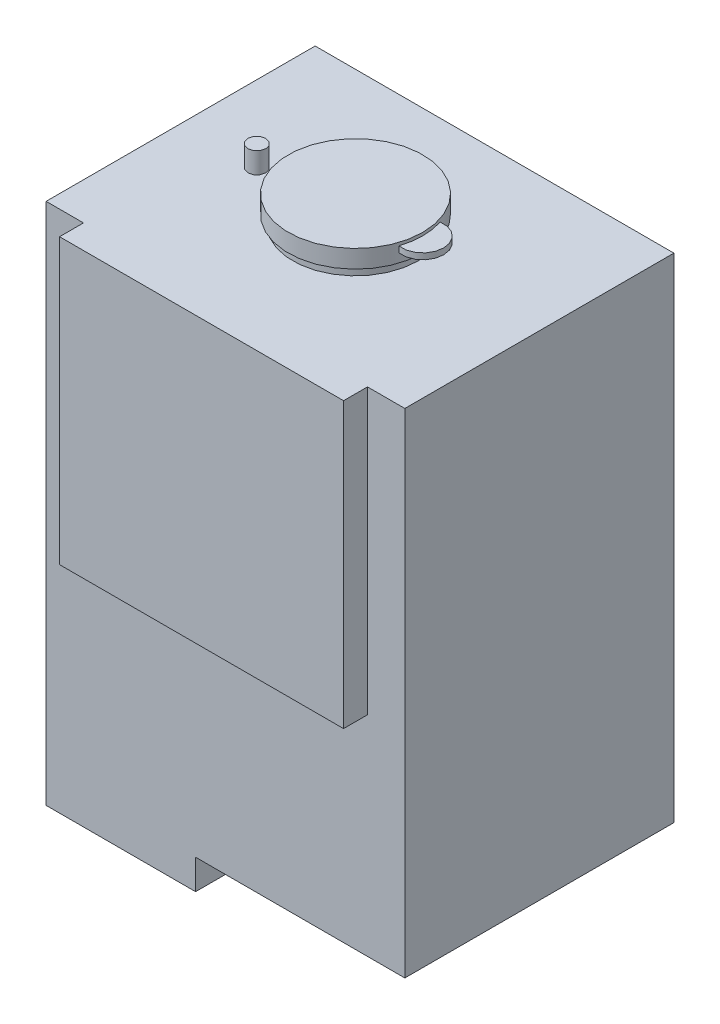
# Autodesk Inventor part: windshield washer
Saved by Autodesk Inventor 2023 (Build 270158030, 158C)
## iProperties
Created: 2023-03-05
Part Number: windshield washer
Material: Generic
Document SubType Name: Modeling
Designer: fatih
Density: 1 g/cm^3
Appearance: Default
Author: fatih
Autodesk Inventor part; units mm, degrees
sketch "Sketch2" plane through (0, 0, 0) normal (0, 0, 1) x (1, 0, 0)
  line L0 (0, 0) -> (70, 0)
  line L1 (70, 0) -> (70, 165)
  line L2 (70, 165) -> (0, 165)
  line L3 (0, 165) -> (0, 0)
  dimension "d0" = 165
  dimension "d1" = 70
  constraints: 8 end point, 2 parallel, 1 horizontal, 1 perpendicular
  measures "d0" distance of L0.end L1.end
  measures "d1" distance of L0.start L0.end
extrude "Extrusion1" add sketch "Sketch2" along normal blind 90
sketch "Sketch6" plane through (0, 0, 0) normal (-1, 0, 0) x (0, 0, 1)
  line L0 (90, 0) -> (90, 165) projected
  line L1 (0, 0) -> (0, 165) projected
  line L2 (90, 165) -> (0, 165)
  line L3 (0, 165) -> (0, 65)
  line L4 (0, 65) -> (90, 65)
  line L5 (90, 65) -> (90, 165)
  dimension "d8" = 100
  constraints: 8 end point, 2 parallel, 1 horizontal, 1 perpendicular, 1 point on line
  measures "d8" distance of L2.end L3.end
extrude "Extrusion3" add sketch "Sketch6" along normal blind 50
sketch "Sketch7" plane through (0, 65, 0) normal (0, -1, 0) x (1, 0, 0)
  line L0 (70, 90) -> (-50, 90) projected
  line L1 (0, 0) -> (0, 90) projected
  line L2 (-50, 90) -> (0, 90)
  line L3 (0, 90) -> (0, 38)
  line L4 (0, 38) -> (-50, 38)
  line L5 (-50, 38) -> (-50, 90)
  dimension "d11" = 52
  constraints: 8 end point, 2 parallel, 1 horizontal, 1 perpendicular, 1 point on line
  measures "d11" distance of L4.end L0.end
extrude "Extrusion4" add sketch "Sketch7" along normal blind 75
sketch "Sketch8" plane through (0, 65, 38) normal (0, 0, -1) x (-1, 0, 0)
  line L0 (0, 0) -> (50, 0) projected
  line L1 (50, 0) -> (29, 0)
  line L2 (29, 0) -> (29, -45)
  line L3 (29, -45) -> (50, -45)
  line L4 (50, -45) -> (50, 0)
  point P0 (0, -65)
  point P1 (29, 0)
  dimension "d14" = 21
  dimension "d15" = 45
  constraints: 8 end point, 2 parallel, 1 horizontal, 1 perpendicular
  measures "d14" distance of L2.end L3.end
  measures "d15" distance of L1.end L2.end
extrude "Extrusion5" add sketch "Sketch8" along normal blind 25
sketch "Sketch9" plane through (0, 0, 90) normal (0, 0, 1) x (1, 0, 0)
  line L0 (70, 165) -> (-50, 165) projected
  line L1 (-50, 165) -> (70, 165)
  line L2 (70, 165) -> (10, 165)
  line L3 (10, 70) -> (57.5, 70)
  line L4 (57.5, 70) -> (-37.5, 70)
  line L5 (-37.5, 70) -> (-37.5, 165)
  line L6 (57.5, 70) -> (57.5, 165)
  point P0 (0, 0)
  dimension "d20" = 95
  dimension "d21" = 95
  constraints: 12 end point, 3 point on line, 2 horizontal, 2 perpendicular, 1 midpoint
  measures "d20" distance of L3.end L4.end
  measures "d21" distance of L3.end L6.end
extrude "Extrusion6" add sketch "Sketch9" along normal blind 8
ref_plane "Work Plane1" through (-48, 65, 2) normal (0, -1, 0) x (1, 0, 0)
sketch "Sketch10" plane through (-48, 65, 2) normal (0, -1, 0) x (1, 0, 0)
  line L0 (21, 34) -> (46, 34) projected
  line L1 (33.5, 34) -> (33.5, 0)
  line L2 (46, 0) -> (0, 0) projected
  circle A0 centre (33.5, 17) radius 12.5
  point P0 (48, -2)
  constraints: 2 end point, 2 midpoint, 1 centre point, 1 point on line, 1 vertical
extrude "Extrusion7" add sketch "Sketch10" along normal blind 70
ref_plane "Work Plane3" through (-48, 165, 5) normal (0, 1, 0) x (1, 0, 0)
sketch "Sketch11" plane through (-48, 165, 5) normal (0, 1, 0) x (1, 0, 0)
  line L0 (113, 0) -> (113, -80) projected
  line L1 (0, -80) -> (0, 0) projected
  circle A0 centre (56.5, -40) radius 21
  point P0 (48, 5)
  dimension "d29" = 42
  constraints: 1 centre point
  measures "d29" diameter of A0
extrude "Extrusion8" add sketch "Sketch11" along normal blind 6
ref_plane "Work Plane2" through (-48, 165, 5) normal (0, 1, 0) x (1, 0, 0)
sketch "Sketch12" plane through (-48, 165, 5) normal (0, 1, 0) x (1, 0, 0)
  circle A0 centre (56.5, -40) radius 21 projected
  line L0 (35.5, -40) -> (26.5, -40)
  circle A1 centre (23.5, -40) radius 3
  point P0 (48, 5)
  dimension "d32" = 9
  constraints: 2 end point, 1 centre point, 1 horizontal, 1 horizontal alignment, 1 other
  measures "d32" distance of L0.start L0.end
extrude "Extrusion9" add sketch "Sketch12" along normal blind 7 contours A1
sketch "Sketch13" plane through (8.5, 171, 45) normal (0, 1, 0) x (1, 0, 0)
  circle A0 centre (0, 0) radius 22.5
  arc A1 (21.4111, -6.9148) -> (21.4111, 6.9148) centre (22.5, 0) ccw
  point P0 (-8.5, 45)
  dimension "d37" = 45
  dimension "d38" = 14
  constraints: 5 point on circle, 2 centre point
  measures "d37" diameter of A0
  measures "d38" diameter of A1
extrude "Extrusion10" add sketch "Sketch13" along normal mid plane 6 contours A0
extrude "Extrusion11" add sketch "Sketch13" along normal blind 2 contours A0 A1
body "Solid1"
